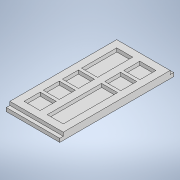
# Autodesk Inventor part: Лого ШП
Saved by Autodesk Inventor 2020 (Build 240168000, 168)
## iProperties
Created: 2021-06-18
Part Number: Лого ШП
Material: Типовые
Document SubType Name: Modeling
Designer: Антон
Density: 1 g/cm^3
Appearance: По умолчанию
Author: Антон
Autodesk Inventor part; units mm, degrees
ref_plane "YZ Plane" through (0, 0, 0) normal (1, 0, 0) x (0, 1, 0)
ref_plane "XZ Plane" through (0, 0, 0) normal (0, 1, 0) x (-1, 0, 0)
ref_plane "XY Plane" through (0, 0, 0) normal (0, 0, 1) x (1, 0, 0)
sketch "Эскиз1" plane through (0, 0, 0) normal (0, 1, 0) x (-1, 0, 0)
  line L0 (0, 0) -> (15, 0)
  line L1 (15, 0) -> (15, -30)
  line L2 (15, -30) -> (0, -30)
  line L3 (0, -30) -> (0, 0)
  line L4 (13, -2) -> (8.5, -2)
  line L5 (8.5, -2) -> (8.5, -6.5)
  line L6 (8.5, -6.5) -> (13, -6.5)
  line L7 (13, -6.5) -> (13, -2)
  line L8 (13, -7.375) -> (8.5, -7.375)
  line L9 (8.5, -7.375) -> (8.5, -11.875)
  line L10 (8.5, -11.875) -> (13, -11.875)
  line L11 (13, -11.875) -> (13, -7.375)
  line L12 (13, -12.75) -> (8.5, -12.75)
  line L13 (8.5, -12.75) -> (8.5, -17.25)
  line L14 (8.5, -17.25) -> (13, -17.25)
  line L15 (13, -17.25) -> (13, -12.75)
  line L16 (13, -18.125) -> (8.5, -18.125)
  line L17 (8.5, -18.125) -> (8.5, -28)
  line L18 (8.5, -28) -> (13, -28)
  line L19 (13, -28) -> (13, -18.125)
  line L20 (6.5, -18.125) -> (2, -18.125)
  line L21 (2, -18.125) -> (2, -22.625)
  line L22 (2, -22.625) -> (6.5, -22.625)
  line L23 (6.5, -22.625) -> (6.5, -18.125)
  line L24 (6.5, -23.5) -> (2, -23.5)
  line L25 (2, -23.5) -> (2, -28)
  line L26 (2, -28) -> (6.5, -28)
  line L27 (6.5, -28) -> (6.5, -23.5)
  line L28 (6.5, -2) -> (2, -2)
  line L29 (2, -2) -> (2, -17.25)
  line L30 (2, -17.25) -> (6.5, -17.25)
  line L31 (6.5, -17.25) -> (6.5, -2)
  line L32 (10.75, -6.5) -> (10.75, -7.375)
  line L33 (10.75, -11.875) -> (10.75, -12.75)
  line L34 (10.75, -17.25) -> (10.75, -18.125)
  line L35 (4.25, -17.25) -> (4.25, -18.125)
  line L36 (4.25, -22.625) -> (4.25, -23.5)
  line L37 (10.75, -2) -> (10.75, 0)
  line L38 (10.75, -28) -> (10.75, -30)
  line L39 (13, -9.625) -> (15, -9.625)
  line L40 (2, -9.625) -> (0, -9.625)
  line L41 (8.5, -9.625) -> (6.5, -9.625)
  dimension "d0" = 15
  dimension "d1" = 30
  dimension "d9" = 2
  constraints: 84 end point, 18 equal length, 16 midpoint, 16 parallel, 11 perpendicular, 9 collinear, 8 horizontal, 4 point on line, 1 vertical
  measures "d0" distance of L1.end L2.end
  measures "d1" distance of L0.end L1.end
  measures "d9" distance of L39.start L39.end
extrude "Выдавливание1" add sketch "Эскиз1" along normal blind 1 contours L0 L37 L4 L5 L6 L32 L8 L9 L41 L31 L28 L29 L40 L3 | L0 L1 L39 L11 L8 L32 L6 L7 L4 L37 | L40 L29 L30 L31 L41 L9 L10 L33 L12 L13 L14 L34 L16 L17 L18 L38 L2 L3 | L1 L2 L38 L18 L19 L16 L34 L14 L15 L12 L33 L10 L11 L39
sketch "Эскиз2" plane through (0, 0, 0) normal (0, -1, 0) x (1, 0, 0)
  line L0 (0, 0) -> (0, -30) projected
  line L1 (-15, 0) -> (0, 0) projected
  line L2 (-15, -30) -> (-15, 0) projected
  line L3 (0, -30) -> (-15, -30) projected
  line L4 (-6.5, -17.25) -> (-2, -17.25) projected
  line L5 (-6.5, -2) -> (-6.5, -17.25) projected
  line L6 (-2, -2) -> (-6.5, -2) projected
  line L7 (-2, -17.25) -> (-2, -2) projected
  line L8 (-2, -28) -> (-2, -23.5) projected
  line L9 (-6.5, -28) -> (-2, -28) projected
  line L10 (-6.5, -23.5) -> (-6.5, -28) projected
  line L11 (-2, -23.5) -> (-6.5, -23.5) projected
  line L12 (-8.5, -12.75) -> (-13, -12.75) projected
  line L13 (-8.5, -17.25) -> (-8.5, -12.75) projected
  line L14 (-13, -17.25) -> (-8.5, -17.25) projected
  line L15 (-13, -12.75) -> (-13, -17.25) projected
  line L16 (-13, -18.125) -> (-13, -28) projected
  line L17 (-8.5, -18.125) -> (-13, -18.125) projected
  line L18 (-8.5, -28) -> (-8.5, -18.125) projected
  line L19 (-13, -28) -> (-8.5, -28) projected
  line L20 (-13, -11.875) -> (-8.5, -11.875) projected
  line L21 (-13, -7.375) -> (-13, -11.875) projected
  line L22 (-8.5, -7.375) -> (-13, -7.375) projected
  line L23 (-8.5, -11.875) -> (-8.5, -7.375) projected
  line L24 (-13, -2) -> (-13, -6.5) projected
  line L25 (-8.5, -2) -> (-13, -2) projected
  line L26 (-8.5, -6.5) -> (-8.5, -2) projected
  line L27 (-13, -6.5) -> (-8.5, -6.5) projected
  line L28 (-2, -22.625) -> (-2, -18.125) projected
  line L29 (-6.5, -22.625) -> (-2, -22.625) projected
  line L30 (-6.5, -18.125) -> (-6.5, -22.625) projected
  line L31 (-2, -18.125) -> (-6.5, -18.125) projected
extrude "Выдавливание2" add sketch "Эскиз2" along normal blind 1 contours L0 L3 L2 L1 | L5 L6 L7 L4 | L9 L10 L11 L8 | L13 L14 L15 L12 | L17 L18 L19 L16 | L21 L22 L23 L20 | L25 L26 L27 L24 | L29 L30 L31 L28
sketch "Эскиз3" plane through (-15, 1, 0) normal (0, 0, 1) x (1, 0, 0)
  line L0 (0, -2) -> (15, -2)
  line L1 (15, -2) -> (15, -1)
  line L2 (15, -1) -> (0, -1)
  line L3 (0, -1) -> (0, -2)
  line L4 (15, -2) -> (15, 0) projected
  line L5 (0, -2) -> (0, 0) projected
  line L6 (15, -2) -> (0, -2) projected
  dimension "d14" = 1
  constraints: 8 end point, 3 collinear, 2 parallel, 1 horizontal, 1 perpendicular
  measures "d14" distance of L0.end L1.end
extrude "Выдавливание3" add sketch "Эскиз3" along normal blind 1
sketch "Эскиз4" plane through (0, 1, -30) normal (0, 0, -1) x (-1, 0, 0)
  line L0 (8.5, -1) -> (13, -1) projected
  line L1 (15, -2) -> (0, -2) projected
  line L2 (0, -2) -> (0, -1) projected
  line L3 (0, -1) -> (15, -1) projected
  line L4 (15, -1) -> (15, -2) projected
extrude "Выдавливание4" add sketch "Эскиз4" along normal blind 1
